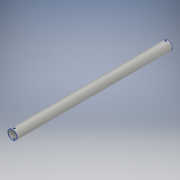
# Autodesk Inventor part: ARM_081_BottomRollerTube
Saved by Autodesk Inventor 2018.3 (Build 223284000, 284)
## iProperties
Created: 2020-02-08
Part Number: ARM_081_BottomRollerTube
Material: Aluminum 6061
Document SubType Name: Modeling
Designer: 22turnmaxw
Density: 2.7 g/cm^3
Appearance: Aluminum - Flat
Mass: 210.708 g
Surface Area: 987.171 cm^2
Volume: 78.04 cm^3
Author: 22turnmaxw
Autodesk Inventor part; units mm, degrees
ref_plane "YZ Plane" through (0, 0, 0) normal (1, 0, 0) x (0, 1, 0)
ref_plane "XY Plane" through (0, 0, 0) normal (0, 0, 1) x (1, 0, 0)
sketch "Sketch1" plane through (0, 0, 0) normal (0, 0, 1) x (1, 0, 0)
  circle A0 centre (0, 0) radius 14.2875
  circle A1 centre (0, 0) radius 15.875
  dimension "d0" = 28.575
  dimension "d1" = 31.75
  constraints: 2 centre point, 2 coincident
  measures "d0" diameter of A0
  measures "d1" diameter of A1
extrude "Extrusion1" add sketch "Sketch1" along normal blind 527.05
ref_plane "Work Plane1" through (0, 25.4, 0) normal (0, 1, 0) x (-1, 0, 0)
sketch "Sketch2" plane through (0, 25.4, 0) normal (0, 1, 0) x (-1, 0, 0)
  line L0 (15.875, 527.05) -> (-15.875, 527.05) projected
  line L1 (-15.875, 0) -> (15.875, 0) projected
  point P0 (0, 0)
  point P1 (0, 6.35)
  point P2 (0, 520.7)
  point P3 (0, 0)
  point P4 (0, 527.05)
  dimension "d5" = 6.35
  dimension "d6" = 6.35
  constraints: 3 vertical alignment, 2 midpoint
  measures "d5" distance from line of L0 point (0, 520.7)
  measures "d6" distance from line of L1 point (0, 6.35)
hole "Hole1" at (0, 25.4, 6.35) at (0, 25.4, 520.7) direction (0, -1, 0) diameter 5.1054 end through all
body "Solid1"
